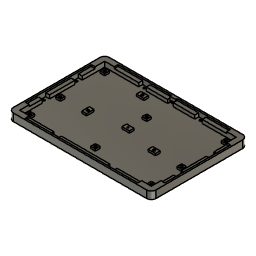
Bottom (Autodesk Fusion 360 design; units mm, degrees)
Autodesk Fusion 360 part; units mm, degrees
sketch "Bottom" plane through (0, 0, 0) normal (0, 0, 1) x (1, 0, 0)
  line L0 (141, -91) -> (-141, -91)
  line L1 (-141, -91) -> (-141, 91)
  line L2 (-141, 91) -> (141, 91)
  line L3 (141, 91) -> (141, -91)
  line L4 (141, -91) -> (-141, 91) construction
  line L5 (-141, -91) -> (141, 91) construction
  line L6 (-153, 103) -> (153, 103)
  line L7 (153, 103) -> (153, -103)
  line L8 (153, -103) -> (-153, -103)
  line L9 (-153, -103) -> (-153, 103)
  line L10 (0, 103) -> (0, -103) construction
  line L11 (-153, 0) -> (153, 0) construction
  line L12 (-149.4, 70.4) -> (-141, 70.4)
  line L13 (-141, 70.4) -> (-141, -70.4)
  line L14 (-141, -70.4) -> (-149.4, -70.4)
  line L15 (-149.4, -70.4) -> (-149.4, 70.4)
  line L16 (-149.4, 0) -> (-141, 0) construction
  line L17 (141, -70.3667) -> (141, 70.4333)
  line L18 (149.4, 70.4333) -> (149.4, -70.3667)
  line L19 (141, 70.4333) -> (149.4, 70.4333)
  line L20 (141, 0.0333) -> (149.4, 0.0333) construction
  line L21 (149.4, -70.3667) -> (141, -70.3667)
  line L22 (-120.4, -91) -> (120.4, -91)
  line L23 (120.4, -91) -> (120.4, -99.4)
  line L24 (120.4, -99.4) -> (-120.4, -99.4)
  line L25 (-120.4, -99.4) -> (-120.4, -91)
  line L26 (0, -99.4) -> (0, -91) construction
  line L27 (-6, 96) -> (6, 96)
  line L28 (6, 96) -> (6, 91)
  line L29 (6, 91) -> (-6, 91)
  line L30 (-6, 91) -> (-6, 96)
  line L31 (0, 96) -> (0, 91) construction
  line L32 (-149.4, 42.9) -> (-141, 42.9)
  line L33 (-141, 42.9) -> (-141, 27.1)
  line L34 (-141, 27.1) -> (-149.4, 27.1)
  line L35 (-149.4, 27.1) -> (-149.4, 42.9)
  line L36 (-149.4, 35) -> (-141, 35) construction
  line L37 (-149.4, -27.1) -> (-141, -27.1)
  line L38 (-149.4, -35) -> (-141, -35) construction
  line L39 (-149.4, -42.9) -> (-149.4, -27.1)
  line L40 (-141, -42.9) -> (-149.4, -42.9)
  line L41 (-141, -27.1) -> (-141, -42.9)
  line L42 (141, 42.9) -> (149.4, 42.9)
  line L43 (141, 35) -> (149.4, 35) construction
  line L44 (141, 27.1) -> (141, 42.9)
  line L45 (149.4, 27.1) -> (141, 27.1)
  line L46 (149.4, 42.9) -> (149.4, 27.1)
  line L47 (141, -27.1) -> (149.4, -27.1)
  line L48 (141, -35) -> (149.4, -35) construction
  line L49 (141, -42.9) -> (141, -27.1)
  line L50 (149.4, -42.9) -> (141, -42.9)
  line L51 (149.4, -27.1) -> (149.4, -42.9)
  line L52 (-52.1, 99.4) -> (-52.1, 91)
  line L53 (-60, 99.4) -> (-60, 91) construction
  line L54 (-67.9, 99.4) -> (-52.1, 99.4)
  line L55 (-67.9, 91) -> (-67.9, 99.4)
  line L56 (-52.1, 91) -> (-67.9, 91)
  line L57 (52.1001, 91) -> (52.1, 99.4)
  line L58 (67.8999, 91) -> (52.1001, 91)
  line L59 (52.1, 99.4) -> (67.9, 99.4)
  line L60 (67.9, 99.4) -> (67.8999, 91)
  line L61 (60, 99.4) -> (60, 91) construction
  line L62 (-67.9, -99.4) -> (-67.9, -91)
  line L63 (-52.1, -99.4) -> (-67.9, -99.4)
  line L64 (-67.9, -91) -> (-52.1, -91)
  line L65 (-52.1, -91) -> (-52.1, -99.4)
  line L66 (-60, -91) -> (-60, -99.4) construction
  line L67 (52.1001, -99.4) -> (52.1, -91)
  line L68 (67.8999, -99.4) -> (52.1001, -99.4)
  line L69 (52.1, -91) -> (67.9, -91)
  line L70 (67.9, -91) -> (67.8999, -99.4)
  line L71 (60, -91) -> (60, -99.4) construction
  line L72 (-120.4, 99.4) -> (-6, 99.4)
  line L73 (-6, 99.4) -> (-6, 91)
  line L74 (-6, 91) -> (-120.4, 91)
  line L75 (-120.4, 91) -> (-120.4, 99.4)
  line L76 (6, 99.4) -> (120.4, 99.4)
  line L77 (120.4, 99.4) -> (120.4, 91)
  line L78 (120.4, 91) -> (6, 91)
  line L79 (6, 91) -> (6, 99.4)
  line L80 (-125, 75) -> (-135, 75)
  line L81 (-135, 75) -> (-135, 85)
  line L82 (-135, 85) -> (-125, 85)
  line L83 (-125, 85) -> (-125, 75)
  line L84 (-125, 75) -> (-135, 85) construction
  line L85 (-135, 75) -> (-125, 85) construction
  line L86 (-125, -10) -> (-125, -20)
  line L87 (-125, -20) -> (-135, -10) construction
  line L88 (-135, -20) -> (-125, -10) construction
  line L89 (-135, -10) -> (-125, -10)
  line L90 (-125, -20) -> (-135, -20)
  line L91 (-135, -20) -> (-135, -10)
  line L92 (-125, -75) -> (-125, -85)
  line L93 (-135, -85) -> (-135, -75)
  line L94 (-135, -85) -> (-125, -75) construction
  line L95 (-125, -85) -> (-135, -85)
  line L96 (-125, -85) -> (-135, -75) construction
  line L97 (-135, -75) -> (-125, -75)
  line L98 (125, -20) -> (135, -10) construction
  line L99 (125, -10) -> (135, -10)
  line L100 (135, 75) -> (125, 85) construction
  line L101 (135, 75) -> (125, 75)
  line L102 (125, 75) -> (135, 85) construction
  line L103 (135, -85) -> (125, -85)
  line L104 (125, 75) -> (125, 85)
  line L105 (135, -10) -> (135, -20)
  line L106 (125, 85) -> (135, 85)
  line L107 (125, -75) -> (135, -75)
  line L108 (125, -85) -> (135, -75) construction
  line L109 (125, -20) -> (125, -10)
  line L110 (125, -85) -> (125, -75)
  line L111 (135, -20) -> (125, -20)
  line L112 (135, -20) -> (125, -10) construction
  line L113 (135, -75) -> (135, -85)
  line L114 (135, 85) -> (135, 75)
  line L115 (135, -85) -> (125, -75) construction
  line L116 (-5, -75) -> (5, -65) construction
  line L117 (5, 35) -> (-5, 45) construction
  line L118 (-5, -65) -> (5, -65)
  line L119 (-5, 35) -> (5, 45) construction
  line L120 (5, -75) -> (-5, -65) construction
  line L121 (5, -75) -> (-5, -75)
  line L122 (-5, -75) -> (-5, -65)
  line L123 (5, 35) -> (-5, 35)
  line L124 (5, -65) -> (5, -75)
  line L125 (-5, 45) -> (5, 45)
  line L126 (5, 45) -> (5, 35)
  line L127 (-5, 35) -> (-5, 45)
  line L128 (0, 45) -> (0, 35) construction
  line L129 (0, -65) -> (0, -75) construction
  line L130 (-53, 71) -> (-37, 71)
  line L131 (-37, 71) -> (-37, 81)
  line L132 (-37, 81) -> (-53, 81)
  line L133 (-53, 81) -> (-53, 71)
  line L134 (-53, 71) -> (-37, 81) construction
  line L135 (-37, 71) -> (-53, 81) construction
  line L136 (78, -19) -> (78, -9)
  line L137 (78, -9) -> (62, -9)
  line L138 (62, -9) -> (62, -19)
  line L139 (62, -19) -> (78, -9) construction
  line L140 (78, -19) -> (62, -9) construction
  line L141 (62, -19) -> (78, -19)
  line L142 (8, -5) -> (-8, -5)
  line L143 (-8, -5) -> (-8, 5)
  line L144 (-8, 5) -> (8, 5)
  line L145 (8, 5) -> (8, -5)
  line L146 (8, -5) -> (-8, 5) construction
  line L147 (-8, -5) -> (8, 5) construction
  line L148 (-70, -19) -> (-80, -19)
  line L149 (-80, -19) -> (-80, -3)
  line L150 (-80, -3) -> (-70, -3)
  line L151 (-70, -3) -> (-70, -19)
  line L152 (-70, -19) -> (-80, -3) construction
  line L153 (-80, -19) -> (-70, -3) construction
  point P0 (-130, 80)
  point P1 (-130, -15)
  point P2 (-130, -80)
  point P3 (130, -15)
  point P4 (130, -80)
  point P5 (130, 80)
  point P6 (0, 40)
  point P7 (0, -70)
  point P8 (-45, 76)
  point P9 (70, -14)
  point P10 (-75, -11)
  dimension "d81" = 282
  dimension "d82" = 182
  dimension "d83" = 12
  dimension "d84" = 12
  dimension "d85" = 12
  dimension "d86" = 12
  dimension "d87" = 8.4
  dimension "d88" = 140.8
  dimension "d89" = 8.4
  dimension "d90" = 140.8
  dimension "d91" = 8.4
  dimension "d92" = 240.8
  dimension "d93" = 12
  dimension "d94" = 5
  dimension "d95" = 15.8
  dimension "d96" = 15.8
  dimension "d97" = 15.8
  dimension "d98" = 15.8
  dimension "d99" = 15.8
  dimension "d100" = 15.8
  dimension "d101" = 15.8
  dimension "d102" = 15.8
  dimension "d103" = 35
  dimension "d104" = 35
  dimension "d105" = 35
  dimension "d106" = 35
  dimension "d107" = 60
  dimension "d108" = 60
  dimension "d109" = 114.4
  dimension "d110" = 8.4
  dimension "d111" = 8.4
  dimension "d112" = 114.4
  dimension "d113" = 10
  dimension "d114" = 10
  dimension "d115" = 10
  dimension "d116" = 10
  dimension "d117" = 10
  dimension "d118" = 10
  dimension "d119" = 10
  dimension "d120" = 10
  dimension "d121" = 10
  dimension "d122" = 10
  dimension "d123" = 10
  dimension "d124" = 10
  dimension "d125" = 10
  dimension "d126" = 10
  dimension "d127" = 10
  dimension "d128" = 10
  dimension "d129" = 130
  dimension "d130" = 80
  dimension "d131" = 130
  dimension "d132" = 15
  dimension "d133" = 130
  dimension "d134" = 80
  dimension "d135" = 130
  dimension "d136" = 80
  dimension "d137" = 130
  dimension "d138" = 15
  dimension "d139" = 130
  dimension "d140" = 80
  dimension "d141" = 70
  dimension "d142" = 40
  dimension "d143" = 60
  dimension "d144" = 60
  dimension "d145" = 16
  dimension "d146" = 10
  dimension "d147" = 16
  dimension "d148" = 10
  dimension "d149" = 70
  dimension "d150" = 14
  dimension "d151" = 45
  dimension "d152" = 76
  dimension "d153" = 16
  dimension "d154" = 10
  dimension "d155" = 10
  dimension "d156" = 16
  dimension "d157" = 75
  dimension "d158" = 11
  constraint horizontal L0
  constraint perpendicular L0 L1
  constraint parallel L0 L2
  constraint parallel L1 L3
  constraint coincident L4 origin
  constraint coincident L5 origin
  constraint horizontal L6
  constraint vertical L7
  constraint horizontal L8
  constraint vertical L9
  constraint midpoint L6 L10.start
  constraint midpoint L8 L10.end
  constraint midpoint L9 L11.start
  constraint midpoint L7 L11.end
  constraint horizontal L12
  constraint vertical L13
  constraint horizontal L14
  constraint vertical L15
  constraint midpoint L15 L16.start
  constraint midpoint L13 L16.end
  constraint collinear L11 L16
  constraint horizontal L19
  constraint vertical L18
  constraint horizontal L21
  constraint vertical L17
  constraint midpoint L20.start L17
  constraint midpoint L20.end L18
  constraint collinear L3 L17
  constraint collinear L1 L13
  constraint horizontal L22
  constraint vertical L23
  constraint horizontal L24
  constraint vertical L25
  constraint midpoint L24 L26.start
  constraint midpoint L22 L26.end
  constraint collinear L10 L26
  constraint collinear L0 L22
  constraint horizontal L27
  constraint vertical L28
  constraint horizontal L29
  constraint vertical L30
  constraint midpoint L27 L31.start
  constraint midpoint L29 L31.end
  constraint collinear L10 L31
  constraint collinear L2 L29
  constraint horizontal L32
  constraint vertical L33
  constraint horizontal L34
  constraint vertical L35
  constraint midpoint L35 L36.start
  constraint midpoint L33 L36.end
  constraint horizontal L37
  constraint vertical L41
  constraint horizontal L40
  constraint vertical L39
  constraint midpoint L38.start L39
  constraint midpoint L38.end L41
  constraint horizontal L42
  constraint vertical L46
  constraint horizontal L45
  constraint vertical L44
  constraint midpoint L43.start L44
  constraint midpoint L43.end L46
  constraint horizontal L47
  constraint vertical L51
  constraint horizontal L50
  constraint vertical L49
  constraint midpoint L48.start L49
  constraint midpoint L48.end L51
  constraint midpoint L53.start L54
  constraint midpoint L53.end L56
  constraint midpoint L61.start L59
  constraint midpoint L61.end L58
  constraint midpoint L66.start L64
  constraint midpoint L66.end L63
  constraint midpoint L71.start L69
  constraint midpoint L71.end L68
  constraint collinear L17 L44
  constraint collinear L18 L46
  constraint collinear L18 L51
  constraint collinear L17 L49
  constraint collinear L1 L41
  constraint collinear L15 L39
  constraint collinear L15 L35
  constraint collinear L13 L33
  constraint collinear L24 L63
  constraint collinear L0 L64
  constraint collinear L24 L68
  constraint collinear L22 L69
  constraint horizontal L72
  constraint vertical L73
  constraint horizontal L74
  constraint vertical L75
  constraint collinear L30 L73
  constraint collinear L2 L74
  constraint horizontal L76
  constraint vertical L77
  constraint horizontal L78
  constraint vertical L79
  constraint collinear L28 L79
  constraint collinear L2 L78
  constraint collinear L59 L76
  constraint collinear L2 L58
  constraint collinear L54 L72
  constraint collinear L2 L56
  constraint horizontal L80
  constraint perpendicular L80 L81
  constraint parallel L80 L82
  constraint parallel L81 L83
  constraint coincident L84 P0
  constraint coincident L85 P0
  constraint horizontal L90
  constraint perpendicular L90 L91
  constraint parallel L89 L90
  constraint parallel L86 L91
  constraint coincident P1 L87
  constraint coincident P1 L88
  constraint horizontal L95
  constraint perpendicular L93 L95
  constraint parallel L95 L97
  constraint parallel L92 L93
  constraint coincident P2 L96
  constraint coincident P2 L94
  constraint horizontal L101
  constraint perpendicular L101 L104
  constraint parallel L101 L106
  constraint parallel L104 L114
  constraint coincident P5 L100
  constraint coincident P5 L102
  constraint horizontal L111
  constraint perpendicular L109 L111
  constraint parallel L99 L111
  constraint parallel L105 L109
  constraint coincident P3 L112
  constraint coincident P3 L98
  constraint horizontal L103
  constraint perpendicular L103 L110
  constraint parallel L103 L107
  constraint parallel L110 L113
  constraint coincident P4 L115
  constraint coincident P4 L108
  constraint horizontal L123
  constraint perpendicular L123 L127
  constraint parallel L123 L125
  constraint parallel L126 L127
  constraint coincident P6 L117
  constraint coincident P6 L119
  constraint horizontal L121
  constraint perpendicular L121 L122
  constraint parallel L118 L121
  constraint parallel L122 L124
  constraint coincident P7 L120
  constraint coincident P7 L116
  constraint midpoint L125 L128.start
  constraint midpoint L123 L128.end
  constraint midpoint L118 L129.start
  constraint midpoint L121 L129.end
  constraint collinear L10 L129
  constraint collinear L10 L128
  constraint horizontal L130
  constraint perpendicular L130 L131
  constraint parallel L130 L132
  constraint parallel L131 L133
  constraint coincident L134 P8
  constraint coincident L135 P8
  constraint horizontal L141
  constraint perpendicular L136 L141
  constraint parallel L137 L141
  constraint parallel L136 L138
  constraint coincident P9 L139
  constraint coincident P9 L140
  constraint horizontal L142
  constraint perpendicular L142 L143
  constraint parallel L142 L144
  constraint parallel L143 L145
  constraint coincident L146 origin
  constraint coincident L147 origin
  constraint horizontal L148
  constraint perpendicular L148 L149
  constraint parallel L148 L150
  constraint parallel L149 L151
  constraint coincident L152 P10
  constraint coincident L153 P10
  measures "d81" distance of L1.end L2.end
  measures "d82" distance of L0.start L2.end
  measures "d83" distance of L2 L6
  measures "d84" distance of L3 L7
  measures "d85" distance of L0 L8
  measures "d86" distance of L1 L9
  measures "d87" distance of L12.start L12.end
  measures "d88" distance of L12.start L14.end
  measures "d89" distance of L18.start L17.end
  measures "d90" distance of L17.end L17.start
  measures "d91" distance of L22.start L24.end
  measures "d92" distance of L23.end L24.end
  measures "d93" distance of L27.start L27.end
  measures "d94" distance of L27.start L29.end
  measures "d95" distance of L32.start L34.end
  measures "d96" distance of L39.start L37.start
  measures "d97" distance of L44.start L42.start
  measures "d98" distance of L49.start L47.start
  measures "d99" distance of L54.start L52.start
  measures "d100" distance of L59.end L57.end
  measures "d101" distance of L64.end L62.end
  measures "d102" distance of L69.end L67.end
  measures "d103" distance of L11 L43
  measures "d104" distance of L11 L48
  measures "d105" distance of L11 L36
  measures "d106" distance of L11 L38
  measures "d107" distance of L10 L66
  measures "d108" distance of L10 L71
  measures "d109" distance of L72.start L72.end
  measures "d110" distance of L72.start L74.end
  measures "d111" distance of L76.end L77.end
  measures "d112" distance of L76.start L76.end
  measures "d113" distance of L80.start L82.end
  measures "d114" distance of L81.end L82.end
  measures "d115" distance of L86.end L86.start
  measures "d116" distance of L87.end L86.start
  measures "d117" distance of L92.start L92.end
  measures "d118" distance of L92.start L93.end
  measures "d119" distance of L100.start L102.end
  measures "d120" distance of L100.end L102.end
  measures "d121" distance of L98.end L105.end
  measures "d122" distance of L98.end L99.start
  measures "d123" distance of L103.start L107.end
  measures "d124" distance of L107.start L107.end
  measures "d125" distance of L119.end L117.start
  measures "d126" distance of L119.end L117.end
  measures "d127" distance of L120.start L116.end
  measures "d128" distance of L118.start L116.end
  measures "d129" distance of L10 P2
  measures "d130" distance of L11 P2
  measures "d131" distance of L10 P1
  measures "d132" distance of L11 P1
  measures "d133" distance of L10 P0
  measures "d134" distance of L11 P0
  measures "d135" distance of L10 P4
  measures "d136" distance of L11 P4
  measures "d137" distance of L10 P3
  measures "d138" distance of L11 P3
  measures "d139" distance of L10 P5
  measures "d140" distance of L11 P5
  measures "d141" distance of L11 P7
  measures "d142" distance of origin P6
  measures "d143" distance of L10 L53
  measures "d144" distance of L10 L61
  measures "d145" distance of L131.end L132.end
  measures "d146" distance of L130.start L132.end
  measures "d147" distance of L136.end L137.end
  measures "d148" distance of L138.end L137.end
  measures "d149" distance of L10 P9
  measures "d150" distance of L11 P9
  measures "d151" distance of L10 P8
  measures "d152" distance of L11 P8
  measures "d153" distance of L143.end L144.end
  measures "d154" distance of L142.start L144.end
  measures "d155" distance of L149.end L150.end
  measures "d156" distance of L148.end L149.end
  measures "d157" distance of L10 P10
  measures "d158" distance of L11 P10
sketch "MidHoles" plane through (0, 0, 0) normal (0, 0, 1) x (1, 0, 0)
  circle A0 centre (0, 0) radius 1.8
  circle A1 centre (0, 0) radius 2.1
  dimension "d159" = 4.2
  dimension "d160" = 3.6
  constraint coincident A0.centre A1.centre
  measures "d159" diameter of A1
  measures "d160" diameter of A0
sketch "Sketch3" plane through (0, 0, 0) normal (0, 0, 1) x (1, 0, 0)
  circle A0 centre (0, 0) radius 1.8
  circle A1 centre (0, 0) radius 3.3
  dimension "d161" = 6.6
  dimension "d162" = 3.6
  constraint coincident A0.centre A1.centre
  constraint concentric A0 A1
  measures "d161" diameter of A1
  measures "d162" diameter of A0
extrude "Extrude1" add sketch "MidHoles" along normal blind 9 and the other way blind -6 makes body 1
extrude "Extrude2" add sketch "MidHoles" along normal blind 9 and the other way blind -4 contours A0 bodies 1
copy_body "Body->Comp1" bodies 1 removing the originals makes body 2 in component "Mid Hole"
extrude "Extrude3" add sketch "Sketch3" along normal blind 4.4 separate body makes body 3
extrude "Extrude4" add sketch "Sketch3" along normal blind 5 contours A0 bodies 3
copy_body "Body->Comp2" bodies 3 removing the originals makes body 4 in component "Side Hole"
extrude "Extrude5" add sketch "Sketch3" along normal blind 4.4 separate body makes body 5
extrude "Extrude6" add sketch "Sketch3" along normal blind 9 contours A0 bodies 5
copy_body "Body->Comp3" bodies 5 removing the originals makes body 6 in component "Middle Hole"
extrude "Extrude7" add sketch "Bottom" along normal blind 16 separate body contours L6 L7 L8 L9 makes body 7
extrude "Extrude8" add sketch "Bottom" along normal blind 12.5 contours L0 L22 L23 L24 L70 | L3 L17 L18 L21 L50 | L0 L22 L24 L65 L67 | L3 L17 L18 L45 L47 | L0 L22 L24 L25 L62 | L3 L17 L18 L19 L42 | L1 L13 L14 L15 L40 | L2 L60 L76 L77 L78 | L1 L13 L15 L34 L37 | L2 L28 L57 L76 L78 L79 | L1 L12 L13 L15 L32 | L2 L30 L52 L72 L73 L74 | L2 L55 L72 L74 L75 bodies 7
extrude "Extrude9" add sketch "Bottom" along normal blind 5 contours L0 L1 L2 L3 L13 L17 L22 L29 L33 L41 L44 L49 L56 L58 L64 L69 L74 L78 | L0 L22 L24 L67 L68 L69 L70 | L3 L17 L18 L47 L49 L50 L51 | L0 L22 L24 L62 L63 L64 L65 | L3 L17 L18 L42 L44 L45 L46 | L1 L13 L15 L37 L39 L40 L41 | L2 L57 L58 L59 L60 L76 L78 | L1 L13 L15 L32 L33 L34 L35 | L2 L27 L28 L29 L30 L73 L79 | L2 L52 L54 L55 L56 L72 L74 bodies 7
extrude "Extrude10" add sketch "Bottom" along normal blind 9 contours L80 L81 L82 L83 | L86 L89 L90 L91 | L92 L93 L95 L97 | L99 L105 L109 L111 | L101 L104 L106 L114 | L103 L107 L110 L113 | L118 L121 L122 L124 | L123 L125 L126 L127 | L130 L131 L132 L133 | L136 L137 L138 L141 | L142 L143 L144 L145 | L148 L149 L150 L151 bodies 7
sketch "Sketch4" plane through (0, 0, 0) normal (0, 1, 0) x (1, 0, 0)
  line L0 (-3, -9) -> (3, -9)
  line L1 (-3, -6) -> (3, -6)
  line L2 (0, -9) -> (0, -6) construction
  line L3 (0, 0) -> (0, -11.7) construction
  line L4 (-12, 0) -> (11.5, 0) construction
  line L5 (-4, -11) -> (4, -11)
  line L6 (-4, -4) -> (4, -4)
  line L7 (0, -11) -> (0, -4) construction
  arc A0 (-4, -4) -> (-4, -11) centre (-4, -7.5) ccw
  arc A1 (4, -11) -> (4, -4) centre (4, -7.5) ccw
  arc A2 (3, -9) -> (3, -6) centre (3, -7.5) ccw
  arc A3 (-3, -6) -> (-3, -9) centre (-3, -7.5) ccw
  dimension "d187" = 6
  dimension "d188" = 3
  dimension "d189" = 9
  dimension "d190" = 8
  dimension "d191" = 8
  dimension "d192" = 2
  dimension "d193" = 2
  constraint horizontal L0
  constraint horizontal L1
  constraint equal L0 L1
  constraint midpoint L0 L2.start
  constraint midpoint L1 L2.end
  constraint coincident L3.start origin
  constraint perpendicular L0 L3
  constraint collinear L2 L3
  constraint horizontal L4
  constraint horizontal L5
  constraint horizontal L6
  constraint midpoint L5 L7.start
  constraint midpoint L6 L7.end
  constraint collinear L3 L7
  constraint tangent L6 A0
  constraint tangent L5 A1
  constraint tangent L0 A2
  constraint tangent L1 A3
  measures "d187" distance of L0.start L0.end
  measures "d188" distance of L0 L1
  measures "d189" distance of L3.start L2.start
  measures "d190" distance of L5.start L5.end
  measures "d191" distance of L6.start L6.end
  measures "d192" distance of L0 L5
  measures "d193" distance of L1 L6
extrude "Extrude13" add sketch "Sketch4" along normal blind 7 and the other way blind -2 separate body makes body 8
extrude "Extrude14" add sketch "Sketch4" along normal blind 5 contours L0 L1 A2 A3 bodies 8
copy_body "Body->Comp5" bodies 8 removing the originals makes body 9 in component "USBC"
combine "Combine4" operation cut target body 7 tool bodies 2 2 2 2 2 2 2 2 2 2 2 body 2 seen with x (1, 0, 0) y (0, 1, 0) z (0, 0, 1) at (0, 40, 0) body 2 seen with x (1, 0, 0) y (0, 1, 0) z (0, 0, 1) at (70, -14, 0) body 2 seen with x (1, 0, 0) y (0, 1, 0) z (0, 0, 1) at (130, -15, 0) body 2 seen with x (1, 0, 0) y (0, 1, 0) z (0, 0, 1) at (-130, 80, 0) body 2 seen with x (1, 0, 0) y (0, 1, 0) z (0, 0, 1) at (-130, -15, 0) body 2 seen with x (1, 0, 0) y (0, 1, 0) z (0, 0, 1) at (130, 80, 0) body 2 seen with x (1, 0, 0) y (0, 1, 0) z (0, 0, 1) at (130, -80, 0) body 2 seen with x (1, 0, 0) y (0, 1, 0) z (0, 0, 1) at (-130, -80, 0) body 2 seen with x (1, 0, 0) y (0, 1, 0) z (0, 0, 1) at (-75, -11, 0) body 2 seen with x (1, 0, 0) y (0, 1, 0) z (0, 0, 1) at (0, -70, 0) body 2 seen with x (1, 0, 0) y (0, 1, 0) z (0, 0, 1) at (-45, 76, 0)
combine "Combine5" operation cut target body 7 tool bodies 6
combine "Combine8" operation cut target body 7 tool bodies 4 4 4 4 4 4 4 4 body 4 seen with x (1, 0, 0) y (0, 1, 0) z (0, 0, 1) at (60, 95, 0) body 4 seen with x (1, 0, 0) y (0, 1, 0) z (0, 0, 1) at (-60, 95, 0) body 4 seen with x (1, 0, 0) y (0, 1, 0) z (0, 0, 1) at (145, 35, 0) body 4 seen with x (1, 0, 0) y (0, 1, 0) z (0, 0, 1) at (-60, -95, 0) body 4 seen with x (1, 0, 0) y (0, 1, 0) z (0, 0, 1) at (60, -95, 0) body 4 seen with x (1, 0, 0) y (0, 1, 0) z (0, 0, 1) at (-145, 35, 0) body 4 seen with x (1, 0, 0) y (0, 1, 0) z (0, 0, 1) at (145, -35, 0) body 4 seen with x (1, 0, 0) y (0, 1, 0) z (0, 0, 1) at (-145, -35, 0)
combine "Combine9" operation cut target body 7 tool bodies 9 body 9 seen with x (1, 0, 0) y (0, 1, 0) z (0, 0, 1) at (0, 96, 0) makes body 10 at (-1, 101, 7)
chamfer "Chamfer2" distance 0.5 angle 45 11 edges at (-131.9579, 80.7594, 9) (-46.9579, 76.7594, 9) (-1.9579, 40.7594, 9) (128.0421, 80.7594, 9) (128.0421, -14.2406, 9) (68.0421, -13.2406, 9) (128.0421, -79.2406, 9) (-1.9579, -69.2406, 9) (-76.9579, -10.2406, 9) (-131.9579, -79.2406, 9) (-131.9579, -14.2406, 9) on bodies 7
fillet "Fillet5" radius 10 4 edges at (-153, -103, 8) (153, -103, 8) (153, 103, 8) (-153, 103, 8) on bodies 7
fillet "Fillet6" radius 2 4 edges at (0, 103, 4) (7.5, 103, 7.5) (0, 103, 11) (-7.5, 103, 7.5) on bodies 7
delete_face "SurfaceDeleteFace1" leaving the opening 4 faces at (-1, 103, 7) (-1, 101.6667, 9) (3.9642, 101.6667, 6.3509) (-4.3673, 101.6667, 8.1169) on bodies 10
delete_face "SurfaceDeleteFace2" leaving the opening 2 faces at (-1, 101.6667, 6) (-1, 101, 7) on bodies 10
sketch "Sketch5" plane through (0, 0, 0) normal (0, 0, 1) x (1, 0, 0)
  circle A0 centre (0, 0) radius 1.8
  circle A1 centre (0, 0) radius 3.3
  line L0 (-3.2265, -0.6925) -> (0.6734, 3.2306)
  line L1 (-0.6734, -3.2306) -> (3.2265, 0.6925)
  line L2 (-0.6925, 3.2265) -> (3.2306, -0.6734)
  line L3 (-3.2306, 0.6734) -> (0.6925, -3.2265)
  line L4 (-2.7659, 1.8) -> (2.7659, 1.8)
  line L5 (-2.7659, -1.8) -> (2.7659, -1.8)
  line L6 (-1.8, -2.7659) -> (-1.8, 2.7659)
  line L7 (1.8, 2.7659) -> (1.8, -2.7659)
  dimension "d220" = 3.6
  dimension "d221" = 6.6
  constraint coincident A0.centre A1.centre
  constraint concentric A0 A1
  constraint tangent A0 L0
  constraint coincident A1 L0.start
  constraint coincident A1 L0.end
  constraint parallel L0 L1
  constraint tangent A0 L1
  constraint coincident A1 L1.end
  constraint coincident A1 L1.start
  constraint tangent A0 L2
  constraint coincident A1 L2.start
  constraint coincident A1 L2.end
  constraint perpendicular L0 L3
  constraint parallel L2 L3
  constraint tangent A0 L3
  constraint coincident A1 L3.start
  constraint coincident A1 L3.end
  constraint horizontal L4
  constraint tangent A0 L4
  constraint coincident A1 L4.start
  constraint coincident A1 L4.end
  constraint horizontal L5
  constraint tangent A0 L5
  constraint coincident A1 L5.start
  constraint coincident A1 L5.end
  constraint vertical L6
  constraint tangent A0 L6
  constraint coincident A1 L6.end
  constraint coincident A1 L6.start
  constraint parallel L6 L7
  constraint tangent A0 L7
  constraint coincident A1 L7.start
  constraint coincident A1 L7.end
  measures "d220" diameter of A0
  measures "d221" diameter of A1
extrude "Extrude18" add sketch "Sketch5" along normal blind 4.4 and the other way blind -2.8 separate body contours L1 L2 L7 | A1 L1 L2 L4 L7 | A1 L1 L2 L5 L7 | A1 L1 L2 | A1 L4 L7 | A1 L5 L7 | L0 L3 L6 | A1 L0 L3 L4 L6 | A1 L4 L6 | A1 L0 L3 L5 L6 | A1 L5 L6 | A1 L0 L3 makes body 11 at (-3.2963, 0.1561, 3.8667) makes body 12 at (3.2852, -0.3119, 3.8667)
extrude "Extrude19" add sketch "Sketch5" along normal blind 4.4 and the other way blind -3.2 contours L0 L2 L4 | A1 L0 L2 L4 L7 | L1 L3 L5 | A1 L1 L3 L5 L7 | A1 L0 L2 L4 L6 | A1 L0 L2 | A1 L1 L3 L5 L6 | A1 L1 L3 bodies 11 12
extrude "Extrude20" add sketch "Sketch5" along normal blind 4.4 and the other way blind -3.6 contours L2 L4 L7 | L3 L5 L6 bodies 11
extrude "Extrude21" add sketch "Sketch5" along normal blind 4.4 and the other way blind -4 contours L1 L5 L7 | L0 L4 L6 bodies 11
copy_body "Body->Comp6" bodies 11 removing the originals makes body 13 in component "HoleFiller"
combine "Combine10" operation add target body 7 tool bodies 13 13 13 13 13 13 13 13 13 body 13 seen with x (1, 0, 0) y (0, 1, 0) z (0, 0, 1) at (145, -35, 0) body 13 seen with x (1, 0, 0) y (0, 1, 0) z (0, 0, 1) at (145, 35, 0) body 13 seen with x (1, 0, 0) y (0, 1, 0) z (0, 0, 1) at (60, 95, 0) body 13 seen with x (1, 0, 0) y (0, 1, 0) z (0, 0, 1) at (-60, 95, 0) body 13 seen with x (1, 0, 0) y (0, 1, 0) z (0, 0, 1) at (-145, 35, 0) body 13 seen with x (1, 0, 0) y (0, 1, 0) z (0, 0, 1) at (-145, -35, 0) body 13 seen with x (1, 0, 0) y (0, 1, 0) z (0, 0, 1) at (-60, -95, 0) body 13 seen with x (1, 0, 0) y (0, 1, 0) z (0, 0, 1) at (0, 0, 0) body 13 seen with x (1, 0, 0) y (0, 1, 0) z (0, 0, 1) at (60, -95, 0)
component "Mid Hole" placed x (1, 0, 0) y (0, 1, 0) z (0, 0, 1) at (130, 80, 0)
component "Mid Hole" placed x (1, 0, 0) y (0, 1, 0) z (0, 0, 1) at (130, -80, 0)
component "Mid Hole" placed x (1, 0, 0) y (0, 1, 0) z (0, 0, 1) at (130, -15, 0)
component "Mid Hole" placed x (1, 0, 0) y (0, 1, 0) z (0, 0, 1) at (-130, 80, 0)
component "Mid Hole" placed x (1, 0, 0) y (0, 1, 0) z (0, 0, 1) at (-130, -15, 0)
component "Mid Hole" placed x (1, 0, 0) y (0, 1, 0) z (0, 0, 1) at (-130, -80, 0)
component "Mid Hole" placed x (1, 0, 0) y (0, 1, 0) z (0, 0, 1) at (0, -70, 0)
component "Mid Hole" placed x (1, 0, 0) y (0, 1, 0) z (0, 0, 1) at (0, 40, 0)
component "Mid Hole" placed x (1, 0, 0) y (0, 1, 0) z (0, 0, 1) at (70, -14, 0)
component "Mid Hole" placed x (1, 0, 0) y (0, 1, 0) z (0, 0, 1) at (-45, 76, 0)
component "Mid Hole" placed x (1, 0, 0) y (0, 1, 0) z (0, 0, 1) at (-75, -11, 0)
component "Side Hole" placed x (1, 0, 0) y (0, 1, 0) z (0, 0, 1) at (145, 35, 0)
component "Side Hole" placed x (1, 0, 0) y (0, 1, 0) z (0, 0, 1) at (145, -35, 0)
component "Side Hole" placed x (1, 0, 0) y (0, 1, 0) z (0, 0, 1) at (-145, 35, 0)
component "Side Hole" placed x (1, 0, 0) y (0, 1, 0) z (0, 0, 1) at (-145, -35, 0)
component "Side Hole" placed x (1, 0, 0) y (0, 1, 0) z (0, 0, 1) at (60, 95, 0)
component "Side Hole" placed x (1, 0, 0) y (0, 1, 0) z (0, 0, 1) at (60, -95, 0)
component "Side Hole" placed x (1, 0, 0) y (0, 1, 0) z (0, 0, 1) at (-60, 95, 0)
component "Side Hole" placed x (1, 0, 0) y (0, 1, 0) z (0, 0, 1) at (-60, -95, 0)
component "Middle Hole" placed x (1, 0, 0) y (0, 1, 0) z (0, 0, 1) at (0, 0, 0)
component "USBC" placed x (1, 0, 0) y (0, 1, 0) z (0, 0, 1) at (0, 96, 0)
component "HoleFiller" placed x (1, 0, 0) y (0, 1, 0) z (0, 0, 1) at (0, 0, 0)
component "HoleFiller" placed x (1, 0, 0) y (0, 1, 0) z (0, 0, 1) at (145, 35, 0)
component "HoleFiller" placed x (1, 0, 0) y (0, 1, 0) z (0, 0, 1) at (145, -35, 0)
component "HoleFiller" placed x (1, 0, 0) y (0, 1, 0) z (0, 0, 1) at (-145, 35, 0)
component "HoleFiller" placed x (1, 0, 0) y (0, 1, 0) z (0, 0, 1) at (-145, -35, 0)
component "HoleFiller" placed x (1, 0, 0) y (0, 1, 0) z (0, 0, 1) at (60, 95, 0)
component "HoleFiller" placed x (1, 0, 0) y (0, 1, 0) z (0, 0, 1) at (-60, 95, 0)
component "HoleFiller" placed x (1, 0, 0) y (0, 1, 0) z (0, 0, 1) at (-60, -95, 0)
component "HoleFiller" placed x (1, 0, 0) y (0, 1, 0) z (0, 0, 1) at (60, -95, 0)
